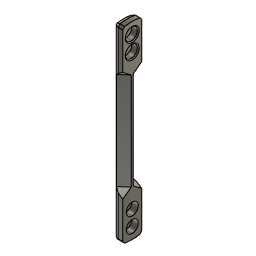
Door Magnet Holder v10 (Autodesk Fusion 360 design; units mm, degrees)
Autodesk Fusion 360 part; units mm, degrees
sketch "Sketch1" plane through (0, 0, 0) normal (1, 0, 0) x (0, 1, 0)
  line L0 (0, 0) -> (10, 0)
  line L1 (10, 0) -> (10, 100)
  line L2 (10, 100) -> (0, 100)
  line L3 (0, 100) -> (0, 0)
  line L4 (5, 0) -> (5, 100) construction
  circle A0 centre (5, 94) radius 3.2
  line L5 (0, 90) -> (10, 90) construction
  circle A1 centre (5, 86) radius 3.2
  arc A2 (0, 0.5051) -> (10, 0.5051) centre (5, 25) ccw
  arc A3 (10, 99.4949) -> (0, 99.4949) centre (5, 75) ccw
  line L6 (0, 50) -> (10, 50) construction
  circle A4 centre (5, 6) radius 3.2
  circle A5 centre (5, 14) radius 3.2
  dimension "d1" = 10
  dimension "d2" = 100
  dimension "d3" = 6.4
  dimension "d4" = 8
  dimension "d11" = 25
  dimension "d20" = 40
  constraint horizontal L0
  constraint vertical L1
  constraint horizontal L2
  constraint vertical L3
  constraint coincident L0.start L3.end
  constraint midpoint L0 L4.start
  constraint midpoint L2 L4.end
  constraint coincident L4 A0.centre
  constraint symmetric A0 L5 A1
  constraint coincident L4.end A3
  constraint coincident L4 A2.centre
  constraint coincident L4.start A2
  constraint equal A2 A3
  constraint coincident L4 A3.centre
  constraint coincident L3 A2.start
  constraint coincident L3 A3.end
  constraint coincident L1 A2.end
  constraint coincident L1 A3.start
  constraint horizontal L5
  constraint coincident L1 L5.end
  constraint coincident L3 L5.start
  constraint midpoint L3 L6.start
  constraint midpoint L1 L6.end
  constraint symmetric A0 L6 A4
  constraint symmetric A1 L6 A5
  measures "d1" distance of L1.end L2.end
  measures "d2" distance of L0.end L1.end
  measures "d3" diameter of A0
  measures "d4" distance of A0.centre A1.centre
  measures "d11" radius of A3
  measures "d20" distance of L5 L6
extrude "Extrude1" add sketch "Sketch1" along normal blind 4.5 contours L1 L3 A2 A3
extrude "Extrude2" add sketch "Sketch1" along normal up to surface (1.1 mm away) contours A0 | A1 | A4 | A5
sketch "Sketch2" plane through (0, 0, 0) normal (0, 0, 1) x (1, 0, 0)
  line L0 (0, 9.5) -> (4.5, 5.5449)
  line L1 (0, 0) -> (0, 10)
  line L2 (0, 0) -> (0, 10)
  line L3 (0, 0) -> (4.5, 0)
  line L4 (4.5, 0) -> (0, 0)
  line L5 (4.5, 8.2) -> (4.5, 1.8)
  line L6 (4.5, 8.2) -> (4.5, 1.8)
  line L7 (4.5, 8.2) -> (4.5, 1.8)
  line L8 (4.5, 8.2) -> (4.5, 1.8)
  line L9 (4.5, 0) -> (4.5, 10)
  line L10 (4.5, 0) -> (4.5, 10)
  line L11 (0, 10) -> (4.5, 10)
  line L12 (4.5, 10) -> (0, 10)
  line L13 (4.5, 5) -> (0, 5) construction
  line L14 (0, 0.5) -> (4.5, 4.4551)
  dimension "d26" = 0.5
  constraint coincident L0.end L9
  constraint coincident L0.start L2
  constraint midpoint L9 L13.start
  constraint midpoint L2 L13.end
  constraint symmetric L0.start L13 L14.start
  constraint symmetric L0.end L13 L14.end
  measures "d26" distance of L0.start L1.end
extrude "Extrude3" cut sketch "Sketch2" along normal mid plane 58 from surface at 50 contours L0 L1 L2 L5 L6 L7 L8 L9 L10 L11 L12 | L1 L2 L3 L4 L5 L6 L7 L8 L9 L10 L14
chamfer "Chamfer1" distance 0.5 angle 45 2 edges at (4.5, 2.0166, 95.1572) (4.5, 2.0166, 87.1572)
chamfer "Chamfer3" distance 1 distance2 1 4 edges at (2.25, 0, 99.4949) (2.25, 10, 99.4949) (2.25, 0, 0.5051) (2.25, 10, 0.5051) measured on face at (3, 7.7908, 99.8437) measured on face at (3, 10, 85.8316) measured on face at (3, 0, 14.1684) measured on face at (3, 4.4407, 0.0063)
chamfer "Chamfer2" distance 2 distance2 1 10 edges at (0, 0, 88.7474) (0, 0, 11.2526) (0, 10, 11.2526) (0, 10, 88.7474) (0, 5, 100) (0, 5, 0) (0, 0.4918, 99.0851) (0, 9.5082, 99.0851) (0, 9.5082, 0.9149) (0, 0.4918, 0.9149) measured on face at (1.5, 0, 91.9966) measured on face at (3, 0, 14.5017) measured on face at (3, 10, 8.0034) measured on face at (3, 10, 85.4983) measured on face at (3, 8.1292, 99.8034) measured on face at (3, 4.5518, 0.004) measured on face at (3, 0.6557, 99.2818) measured on face at (3, 9.6721, 98.8884) measured on face at (1.5, 9.6721, 1.1116) measured on face at (1.5, 0.6557, 0.7182)
chamfer "Chamfer4" distance 3.3 angle 45 4 edges at (2.4313, 7.3631, 21) (2.4313, 7.3631, 79) (2.4313, 2.6369, 21) (2.4313, 2.6369, 79)
